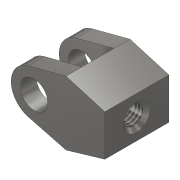
# Autodesk Inventor part: 05.01.001
Saved by Autodesk Inventor 2019.3 (Build 233278000, 278)
## iProperties
Created: 2018-07-09
Part Number: 05.01.001
Material: Сталь, углеродистая
Document SubType Name: Modeling
Designer: MSI-PC
Mass: 120.632 g
Surface Area: 59.0162 cm^2
Volume: 15.3671 cm^3
Density: 7.85 g/cm^3
Appearance: С умеренной полировкой
Description: Вилка
Author: MSI-PC
Autodesk Inventor part; units mm, degrees
ref_plane "YZ Plane" through (0, 0, 0) normal (1, 0, 0) x (0, 1, 0)
ref_plane "XZ Plane" through (0, 0, 0) normal (0, 1, 0) x (-1, 0, 0)
ref_plane "XY Plane" through (0, 0, 0) normal (0, 0, 1) x (1, 0, 0)
sketch "Эскиз1" plane through (0, 0, 0) normal (0, 0, 1) x (1, 0, 0)
  line L0 (-16.5314, 9.6743) -> (0, 14)
  line L1 (0, 14) -> (17, 9)
  line L2 (17, 9) -> (17, 1.7034)
  line L3 (-67.604, 0) -> (31.1007, 0) projected
  line L4 (-16.5314, -9.6743) -> (0, -14)
  line L5 (0, -14) -> (17, -9)
  line L6 (17, -9) -> (17, 1.7034)
  arc A0 (-16.5314, 9.6743) -> (-16.5314, -9.6743) centre (-14, 0) ccw
  point P0 (0, 0)
  point P1 (-53.5033, 0)
  dimension "d0" = 10
  dimension "d1" = 31
  dimension "d2" = 28
  dimension "d3" = 14
  dimension "d4" = 18
  constraints: 12 end point, 3 vertical alignment, 2 point on circle, 2 point on line, 2 tangent, 1 centre point, 1 horizontal alignment, 1 vertical, 1 other
  measures "d0" radius of A0
  measures "d1" distance from line of L6 A0.centre
  measures "d2" distance of L4.end L0.end
  measures "d3" distance of point (0, 0) A0.centre
  measures "d4" distance of L5.end L1.end
extrude "Выдавливание1" add sketch "Эскиз1" along normal mid plane 28
sketch "Эскиз2" plane through (0, 0, 0) normal (0, 1, 0) x (-1, 0, 0)
  line L0 (0, 7) -> (24, 7)
  line L1 (24, 7) -> (24, -7)
  line L2 (24, -7) -> (0, -7)
  line L3 (0, -7) -> (0, 7)
  line L4 (24, -14) -> (24, 14) projected
  point P0 (0, 0)
  point P1 (0, 0)
  dimension "d7" = 14
  constraints: 8 end point, 2 parallel, 1 coincident, 1 collinear, 1 horizontal, 1 midpoint, 1 perpendicular
  measures "d7" distance of L0.end L1.end
extrude "Выдавливание2" cut sketch "Эскиз2" along normal through all both and the other way through all
sketch "Эскиз3" plane through (0, 0, 14) normal (0, 0, 1) x (1, 0, 0)
  arc A0 (-16.5314, 9.6743) -> (-16.5314, -9.6743) centre (-14, 0) ccw projected
  point P0 (0, 0)
  constraints: 1 coincident
hole "Отверстие1" at (-14, 0, 14) direction (0, 0, -1) diameter 12 end through all
sketch "Эскиз4" plane through (17, -9, 14) normal (1, 0, 0) x (0, 0, -1)
  line L0 (28, 18) -> (0, 18) projected
  line L1 (28, 18) -> (28, 0) projected
  point P0 (14, 9)
  point P1 (14, 9)
  dimension "d17" = 9
  dimension "d18" = 14
  measures "d17" distance from line of L0 point (14, 9)
  measures "d18" distance from line of L1 point (14, 9)
hole "Отверстие2" at (17, 0, 0) direction (-1, 0, 0) diameter 8.376 end through all thread size "M10x1.5" class "6H" standard "ISO Metric profile"
chamfer "Фаска1" distance 1.6 angle 45 1 edges at (17, 0, 4.188)
